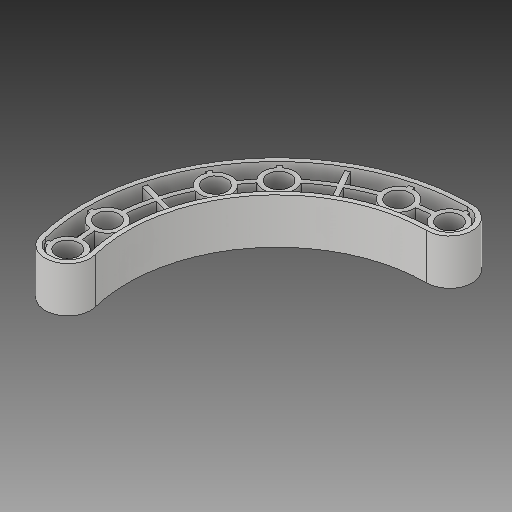
# Autodesk Inventor part: Curved_beam_6h
Saved by Autodesk Inventor 2019.3 (Build 233278000, 278)
## iProperties
Created: 2019-01-29
Part Number: Curved_beam_6h
Material: Generic
Document SubType Name: Modeling
Designer: Varga Daniel
Density: 1 g/cm^3
Appearance: Default
Author: Varga Daniel
Autodesk Inventor part; units mm, degrees
ref_plane "YZ Plane" through (0, 0, 0) normal (1, 0, 0) x (0, 1, 0)
ref_plane "XZ Plane" through (0, 0, 0) normal (0, 1, 0) x (-1, 0, 0)
ref_plane "XY Plane" through (0, 0, 0) normal (0, 0, 1) x (1, 0, 0)
derived "Base_part.ipt"
sketch "Beam_sketch" plane through (0, 0, 0) normal (0, 1, 0) x (-1, 0, 0)
  line L0 (5, 0) -> (25, 0)
  line L1 (30, 5) -> (30, 25)
  line L2 (25, 30) -> (5, 30)
  line L3 (0, 25) -> (0, 5)
  line L4 (5, 29) -> (25, 29)
  line L5 (29, 25) -> (29, 5)
  line L6 (25, 1) -> (5, 1)
  line L7 (1, 5) -> (1, 25)
  circle A0 centre (5, 5) radius 2.5
  circle A1 centre (5, 5) radius 3.5
  arc A2 (25, 0) -> (30, 5) centre (25, 5) ccw
  arc A3 (30, 25) -> (25, 30) centre (25, 25) ccw
  arc A4 (5, 30) -> (0, 25) centre (5, 25) ccw
  arc A5 (0, 5) -> (5, 0) centre (5, 5) ccw
  arc A6 (1, 5) -> (5, 1) centre (5, 5) ccw
  arc A7 (5, 29) -> (1, 25) centre (5, 25) ccw
  arc A8 (29, 25) -> (25, 29) centre (25, 25) ccw
  arc A9 (25, 1) -> (29, 5) centre (25, 5) ccw
  line L8 (49.1041, 15) -> (-27.081, 15) construction
  circle A10 centre (15, 5) radius 2.5
  circle A11 centre (15, 5) radius 3.5
  line L9 (31.1478, 10) -> (-2.4877, 10) construction
  line L10 (-2.8604, 5) -> (35.495, 5) construction
  line L11 (5, -2.5736) -> (5, 36.7522) construction
  line L12 (15, -1.4978) -> (15, 34.8784) construction
  line L13 (18.4641, 5.5) -> (21.5359, 5.5)
  line L14 (18.4641, 4.5) -> (21.5359, 4.5)
  line L15 (1.5359, 5.5) -> (1, 5.5)
  line L16 (1.5359, 4.5) -> (1.0314, 4.5)
  line L17 (28.9686, 4.5) -> (8.4641, 4.5)
  line L18 (29, 5.5) -> (8.4641, 5.5)
  line L19 (4.5, 1.5359) -> (4.5, 1.0314)
  line L20 (5.5, 1.5359) -> (5.5, 1)
  line L21 (29, 10.5) -> (1, 10.5)
  line L22 (29, 9.5) -> (1, 9.5)
  line L23 (4.5, 28.9686) -> (4.5, 10.5)
  line L24 (4.5, 9.5) -> (4.5, 8.4641)
  line L25 (5.5, 29) -> (5.5, 10.5)
  line L26 (5.5, 9.5) -> (5.5, 8.4641)
  point P0 (0, 0)
  point P1 (30, 30)
  point P2 (0, 30)
sketch "Sketch2" plane through (0, 0, 0) normal (0, 1, 0) x (-1, 0, 0)
  arc A0 (0, -33) -> (31.9814, 8.1357) centre (0, 0) ccw
  arc A1 (0, -38) -> (36.8271, 9.3684) centre (0, 0) ccw construction
  arc A2 (0, -43) -> (41.6727, 10.6011) centre (0, 0) ccw
  line L0 (0, -33) -> (0, -43) construction
  line L1 (31.9814, 8.1357) -> (41.6727, 10.6011) construction
  arc A3 (0, -34) -> (32.9505, 8.3823) centre (0, 0) ccw
  arc A4 (0, -42) -> (40.7036, 10.3546) centre (0, 0) ccw
  circle A5 centre (0, -38) radius 3.5
  circle A6 centre (9.9131, -36.6842) radius 3.5
  arc A7 (0, -33) -> (0, -43) centre (0, -38) ccw
  arc A8 (0, -34) -> (0, -42) centre (0, -38) ccw
  arc A9 (41.6727, 10.6011) -> (31.9814, 8.1357) centre (36.8271, 9.3684) ccw
  arc A10 (40.7036, 10.3546) -> (32.9505, 8.3823) centre (36.8271, 9.3684) ccw
  circle A11 centre (36.8271, 9.3684) radius 3.5
  circle A12 centre (37.9958, -0.563) radius 3.5
  circle A13 centre (26.6702, -27.0684) radius 3.5
  circle A14 centre (32.8081, -19.1737) radius 3.5
  line L2 (0, 0) -> (33.9474, -26.3927) construction
  arc A15 (36.2999, 12.8285) -> (36.1273, 13.3067) centre (0, 0) ccw
  arc A16 (35.342, 12.5377) -> (35.171, 13.0095) centre (0, 0) ccw
  arc A17 (37.3889, 2.8839) -> (37.037, 5.8747) centre (0, 0) ccw
  arc A18 (38.3895, 2.9147) -> (38.0174, 6.077) centre (0, 0) ccw
  arc A19 (34.861, -16.3389) -> (38.2863, -4.051) centre (0, 0) ccw
  arc A20 (33.9746, -15.8738) -> (37.2871, -3.9905) centre (0, 0) ccw
  arc A21 (28.6572, -24.1871) -> (30.5056, -21.8096) centre (0, 0) ccw
  arc A22 (29.3916, -24.8674) -> (31.3459, -22.3536) centre (0, 0) ccw
  arc A23 (13.06, -35.1523) -> (23.7598, -29.0124) centre (0, 0) ccw
  arc A24 (13.3649, -36.1058) -> (24.4292, -29.7568) centre (0, 0) ccw
  arc A25 (-3.937, -37.2928) -> (-3.4376, -37.3421) centre (0, 0) ccw
  arc A26 (3.4376, -37.3421) -> (6.4229, -36.9459) centre (0, 0) ccw
  arc A27 (-3.9893, -38.2928) -> (-3.4832, -38.3421) centre (0, 0) ccw
  arc A28 (3.4832, -38.3421) -> (6.6397, -37.9231) centre (0, 0) ccw
  line L3 (0, -38) -> (0, 0) construction
  line L4 (9.9131, -36.6842) -> (0, 0) construction
  line L5 (26.6702, -27.0684) -> (0, 0) construction
  line L6 (32.8081, -19.1737) -> (0, 0) construction
  line L7 (37.9958, -0.563) -> (0, 0) construction
  line L8 (36.8271, 9.3684) -> (0, 0) construction
  line L9 (8.3859, -32.9496) -> (8.5267, -33.4705)
  line L10 (10.334, -40.1588) -> (10.4731, -40.6733)
  line L11 (9.3513, -32.6887) -> (9.4921, -33.2096)
  line L12 (11.2994, -39.8979) -> (11.4384, -40.4124)
  line L13 (0.5, -33.9963) -> (0.5, -34.5359)
  line L14 (0.5, -41.4641) -> (0.5, -41.997)
  line L15 (-0.5, -41.9686) -> (-0.5, -41.4641)
  line L16 (-0.5, -34.5359) -> (-0.5, -34.0314)
  circle A29 centre (0, -38) radius 2.5
  circle A30 centre (15, 5) radius 2.5 construction
  circle A31 centre (15, 5) radius 3.5 construction
  line L17 (18.4641, 5.5) -> (21.5359, 5.5) construction
  line L18 (-2.8604, 5) -> (35.495, 5) construction
  line L19 (18.4641, 4.5) -> (21.5359, 4.5) construction
  line L20 (1, 5) -> (1, 25) construction
  line L21 (0, 25) -> (0, 5) construction
  circle A32 centre (9.9131, -36.6842) radius 2.5
  circle A33 centre (26.6702, -27.0684) radius 2.5
  circle A34 centre (32.8081, -19.1737) radius 2.5
  circle A35 centre (37.9958, -0.563) radius 2.5
  circle A36 centre (36.8271, 9.3684) radius 2.5
  line L22 (23.5041, -24.5674) -> (23.8828, -24.9517)
  line L23 (29.8317, -29.5647) -> (29.4577, -29.185)
  line L24 (24.5951, -24.2499) -> (24.2164, -23.8655)
  line L25 (28.7454, -29.8869) -> (29.1194, -30.2665)
  line L26 (29.0992, -17.5852) -> (29.565, -17.8575)
  line L27 (35.5466, -21.3532) -> (36.0067, -21.6221)
  line L28 (36.5113, -20.7587) -> (36.0512, -20.4899)
  line L29 (30.0696, -16.9941) -> (29.6037, -16.7218)
  line L30 (33.9852, -1.0037) -> (34.5247, -1.0117)
  line L31 (41.4521, -1.1143) -> (41.985, -1.1222)
  line L32 (34, -0.0038) -> (34.5395, -0.0118)
  line L33 (41.467, -0.1144) -> (41.9998, -0.1223)
  line L34 (40.5499, 10.8314) -> (40.061, 10.707)
  line L35 (33.3466, 8.999) -> (32.8577, 8.8746)
  line L36 (33.0702, 7.8968) -> (33.5932, 8.0298)
  line L37 (40.3075, 9.7379) -> (40.824, 9.8693)
  line L38 (36.6045, -10.2036) -> (0, 0) construction
  line L39 (40.589, -10.7952) -> (37.2172, -9.8553)
  line L40 (36.2539, -9.5868) -> (32.8821, -8.6469)
  line L41 (32.6136, -9.6101) -> (35.9854, -10.55)
  line L42 (36.9487, -10.8186) -> (40.3205, -11.7584)
  line L43 (17.354, -29.2376) -> (19.0961, -32.2736)
  line L44 (19.5939, -33.1411) -> (21.336, -36.177)
  line L45 (16.4866, -29.7353) -> (18.2288, -32.7713)
  line L46 (18.7265, -33.6388) -> (20.4687, -36.6747)
  line L47 (20.9038, -36.4284) -> (0, 0) construction
  dimension "d7" = 7
  dimension "d8" = 7
  dimension "d16" = 7
  dimension "d17" = 7
  dimension "d22" = 7
  dimension "d23" = 7
  dimension "d0" = 33
  dimension "d3" = 10
  dimension "d4" = 5
  dimension "d5" = 1
  dimension "d6" = 1
  dimension "d14" = 10
  dimension "d15" = 4
  dimension "d21" = 10
  dimension "d24" = 10
  dimension "d28" = 5
  dimension "d34" = 1
  dimension "d35" = 0.5
  dimension "d37" = 1
  dimension "d38" = 1
  dimension "d39" = 5
  dimension "d40" = 5
  dimension "d41" = 7
  dimension "d42" = 5
  dimension "d43" = 5
  dimension "d44" = 5
  dimension "d45" = 5
  dimension "d46" = 5
  dimension "d48" = 1
  dimension "d49" = 1
  dimension "d51" = 1
  dimension "d53" = 1
  dimension "d54" = 29.454
  dimension "d55" = 14.727
  dimension "d57" = 1
  dimension "d74" = 1
  dimension "d75" = 60
  constraints: 86 end point, 66 point on circle, 27 centre point, 27 parallel, 16 collinear, 14 coincident, 12 concentric, 7 point on line, 2 midpoint, 2 vertical, 1 tangent, 111 other
  measures "d0" radius of A0
  measures "d3" radial gap between concentric circles of A2 A0
  measures "d4" radial gap between concentric circles of A1 A0
  measures "d14" distance of A1.start L4.start
  measures "d15" radius of A8
  measures "d21" distance of A9.centre L7.start
  measures "d24" distance of L5.start L6.start
  measures "d28" distance from line of L6.start L2
  measures "d34" radial gap between concentric circles of A26 A28
  measures "d35" radial gap between concentric circles of A1 A28
  measures "d37" distance between parallel lines of L16 L13
  measures "d38" distance between parallel lines of L9 L11
  measures "d39" diameter of A29
  measures "d40" diameter of A30
  measures "d41" diameter of A31
  measures "d42" diameter of A32
  measures "d43" diameter of A33
  measures "d44" diameter of A34
  measures "d45" diameter of A35
  measures "d46" diameter of A36
  measures "d48" distance between parallel lines of L24 L22
  measures "d49" distance between parallel lines of L29 L26
  measures "d51" distance between parallel lines of L32 L30
  measures "d53" distance between parallel lines of L35 L36
  measures "d54" angle of L7 L6
  measures "d55" angle of L38 L6
  measures "d57" distance between parallel lines of L40 L41
  measures "d74" distance of L45.start L43.start
  measures "d75" distance of A1.end L3.start
extrude "Extrusion1" add sketch "Sketch2" along normal blind 5 contours A0 A9 A2 A7
extrude "Extrusion2" add sketch "Sketch2" against normal blind 5 contours A0 A9 A2 A7
extrude "Extrusion3" add sketch "Sketch2" along normal blind 4.2 contours A3 L13 A5 L16 A8 | A3 L11 A6 L9 | A5 | A25 A5 A27 A8 | A6 | A26 A6 A28 A5 | A3 L43 A23 L45 | L15 A5 L14 A4 A8 | A23 A13 A24 A6 | A3 L24 A13 L22 | A6 L12 A4 L10 | A13 | A24 L44 A4 L46 | A3 L29 A14 L26 | A14 | A21 A14 A22 A13 | A13 L23 A4 L25 | A3 L40 A20 L41 | A20 A12 A19 A14 | A3 L32 A12 L30 | A14 L28 A4 L27 | A12 | A19 L39 A4 L42 | A3 A10 L35 A11 L36 | A11 | A17 A11 A18 A12 | A12 L33 A4 L31 | A10 A15 A11 A16 | L37 A11 L34 A10 A4
extrude "Extrusion4" add sketch "Sketch2" against normal blind 4.2 contours A3 L13 A5 L16 A8 | A3 L11 A6 L9 | A5 | A25 A5 A27 A8 | A6 | A26 A6 A28 A5 | A3 L43 A23 L45 | L15 A5 L14 A4 A8 | A23 A13 A24 A6 | A3 L24 A13 L22 | A6 L12 A4 L10 | A13 | A24 L44 A4 L46 | A3 L29 A14 L26 | A14 | A21 A14 A22 A13 | A13 L23 A4 L25 | A3 L40 A20 L41 | A20 A12 A19 A14 | A3 L32 A12 L30 | A14 L28 A4 L27 | A12 | A19 L39 A4 L42 | A3 A10 L35 A11 L36 | A11 | A17 A11 A18 A12 | A12 L33 A4 L31 | A10 A15 A11 A16 | L37 A11 L34 A10 A4
extrude "Extrusion5" add sketch "Sketch2" along normal blind 0.5 contours A3 L9 A6 A26 A5 L13 | L16 A5 A25 A8 | A3 L45 A23 A6 L11 | A27 A5 L15 A8 | A3 L22 A13 A23 L43 | A6 L10 A4 L14 A5 A28 | A24 L46 A4 L12 A6 | A3 L26 A14 A21 A13 L24 | A13 L25 A4 L44 A24 | A3 L41 A20 A14 L29 | A22 A14 L27 A4 L23 A13 | A3 L30 A12 A20 L40 | A19 L42 A4 L28 A14 | A3 L36 A11 A17 A12 L32 | A12 L31 A4 L39 A19 | A10 A16 A11 L35 | A18 A11 L37 A4 L33 A12 | A10 L34 A11 A15
extrude "Extrusion6" add sketch "Sketch2" against normal blind 0.5 contours A3 L9 A6 A26 A5 L13 | L16 A5 A25 A8 | A3 L45 A23 A6 L11 | A27 A5 L15 A8 | A3 L22 A13 A23 L43 | A6 L10 A4 L14 A5 A28 | A24 L46 A4 L12 A6 | A3 L26 A14 A21 A13 L24 | A13 L25 A4 L44 A24 | A3 L41 A20 A14 L29 | A22 A14 L27 A4 L23 A13 | A3 L30 A12 A20 L40 | A19 L42 A4 L28 A14 | A3 L36 A11 A17 A12 L32 | A12 L31 A4 L39 A19 | A10 A16 A11 L35 | A18 A11 L37 A4 L33 A12 | A10 L34 A11 A15
equation "\"d7\" = d41"
equation "\"d8\" = d7"
equation "\"d16\" = d7"
equation "\"d17\" = d7"
equation "\"d22\" = d7"
equation "\"d23\" = d7"
equation "\"d4\" = 0.5 * d3"
equation "\"d5\" = Wall_thickness"
equation "\"d6\" = Wall_thickness"
equation "\"d28\" = 0.5 * d24"
equation "\"d34\" = Inner_route_thickness"
equation "\"d35\" = 0.5 * d34"
equation "\"d37\" = Inner_route_thickness"
equation "\"d38\" = d37"
equation "\"d39\" = d40"
equation "\"d42\" = d39"
equation "\"d43\" = d39"
equation "\"d44\" = d39"
equation "\"d45\" = d39"
equation "\"d46\" = d39"
equation "\"d48\" = d37"
equation "\"d49\" = d37"
equation "\"d30\" = Inner_route_thickness"
equation "\"d31\" = 0.5 * d30"
equation "\"d32\" = Inner_route_thickness"
equation "\"d33\" = 0.5 * d32"
equation "\"d47\" = d37"
equation "\"Wall_thickness\" = 1"
equation "\"Inner_route_thickness\" = 1"
body "Solid1"
